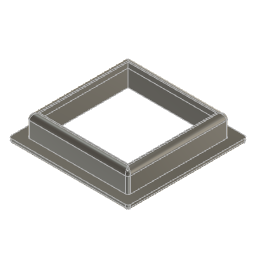
ECM Button Outer v2 (Autodesk Fusion 360 design; units mm, degrees)
Autodesk Fusion 360 part; units mm, degrees
sketch "Sketch1" plane through (0, 0, 0) normal (0, 0, 1) x (1, 0, 0)
  line L0 (9.75, -9.75) -> (-9.75, -9.75)
  line L1 (-9.75, -9.75) -> (-9.75, 9.75)
  line L2 (-9.75, 9.75) -> (9.75, 9.75)
  line L3 (9.75, 9.75) -> (9.75, -9.75)
  line L4 (9.75, -9.75) -> (-9.75, 9.75) construction
  line L5 (-9.75, -9.75) -> (9.75, 9.75) construction
  line L6 (11.5, 11.5) -> (-11.5, 11.5)
  line L7 (-11.5, 11.5) -> (-11.5, -11.5)
  line L8 (-11.5, -11.5) -> (11.5, -11.5)
  line L9 (11.5, -11.5) -> (11.5, 11.5)
  line L10 (11.5, 11.5) -> (-11.5, -11.5) construction
  line L11 (-11.5, 11.5) -> (11.5, -11.5) construction
  line L12 (9.25, -9.25) -> (-9.25, -9.25)
  line L13 (-9.25, -9.25) -> (-9.25, 9.25)
  line L14 (-9.25, 9.25) -> (9.25, 9.25)
  line L15 (9.25, 9.25) -> (9.25, -9.25)
  line L16 (9.25, -9.25) -> (-9.25, 9.25) construction
  line L17 (-9.25, -9.25) -> (9.25, 9.25) construction
  dimension "d1" = 19.5
  dimension "d2" = 19.5
  dimension "d3" = 23
  dimension "d4" = 23
  dimension "d5" = 18.5
  dimension "d6" = 18.5
  constraint horizontal L0
  constraint perpendicular L0 L1
  constraint parallel L0 L2
  constraint parallel L1 L3
  constraint coincident L4 origin
  constraint coincident L5 origin
  constraint horizontal L6
  constraint perpendicular L6 L7
  constraint parallel L6 L8
  constraint parallel L7 L9
  constraint coincident L10 origin
  constraint coincident L11 origin
  constraint horizontal L12
  constraint perpendicular L12 L13
  constraint parallel L12 L14
  constraint parallel L13 L15
  constraint coincident L16 origin
  constraint coincident L17 origin
  measures "d1" distance of L1.end L2.end
  measures "d2" distance of L0.end L1.end
  measures "d3" distance of L7.end L8.end
  measures "d4" distance of L6.end L7.end
  measures "d5" distance of L13.end L14.end
  measures "d6" distance of L12.end L13.end
extrude "Extrude1" add sketch "Sketch1" along normal blind 1 contours L0 L1 L2 L3 | L6 L7 L8 L9 makes body 1
extrude "Extrude2" add sketch "Sketch1" along normal blind 5 contours L12 L13 L14 L15 bodies 1
sketch "Sketch2" plane through (0, 0, 5) normal (0, 0, 1) x (-1, 0, 0)
  line L0 (-9.25, -9.25) -> (9.25, -9.25)
  line L1 (9.25, -9.25) -> (9.25, 9.25)
  line L2 (9.25, 9.25) -> (-9.25, 9.25)
  line L3 (-9.25, 9.25) -> (-9.25, -9.25)
  line L4 (8.5, 8.5) -> (-8.5, 8.5)
  line L5 (-8.5, 8.5) -> (-8.5, -8.5)
  line L6 (-8.5, -8.5) -> (8.5, -8.5)
  line L7 (8.5, -8.5) -> (8.5, 8.5)
  line L8 (8.5, 8.5) -> (-8.5, -8.5) construction
  line L9 (-8.5, 8.5) -> (8.5, -8.5) construction
  dimension "d11" = 17
  dimension "d12" = 17
  constraint horizontal L4
  constraint perpendicular L4 L5
  constraint parallel L4 L6
  constraint parallel L5 L7
  constraint coincident L8 origin
  constraint coincident L9 origin
  measures "d11" distance of L5.end L6.end
  measures "d12" distance of L4.end L5.end
extrude "Extrude3" cut sketch "Sketch2" against normal blind 10 contours L4 L5 L6 L7 bodies 1
extrude "Extrude4" cut sketch "Sketch1" along normal blind 4 contours L12 L13 L14 L15 bodies 1 makes body 2 at (-2.8333, 9, 4)
extrude "Extrude5" add sketch "Sketch1" along normal blind 5 contours L0 L1 L2 L3 bodies 1 2
fillet "Fillet1" radius 0.5 12 edges at (-9.75, -9.75, 3) (-9.75, 9.75, 3) (9.75, 9.75, 3) (9.75, -9.75, 3) (11.5, 11.5, 0.5) (-11.5, 11.5, 0.5) (11.5, -11.5, 0.5) (-11.5, -11.5, 0.5) (0, -11.5, 0) (11.5, 0, 0) (0, 11.5, 0) (-11.5, 0, 0) on bodies 1
fillet "Fillet2" radius 1 8 edges at (9.6036, 9.6036, 5) (0, 9.75, 5) (-9.6036, 9.6036, 5) (-9.75, 0, 5) (-9.6036, -9.6036, 5) (0, -9.75, 5) (9.6036, -9.6036, 5) (9.75, 0, 5) on bodies 1
